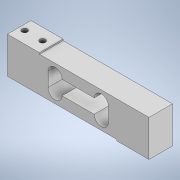
# Autodesk Inventor part: load_cell
Saved by Autodesk Inventor 2022.3 (Build 263350000, 350)
## iProperties
Created: 2022-01-31
Part Number: load_cell
Material: Generic
Document SubType Name: Modeling
Designer: Martijn
Density: 1 g/cm^3
Appearance: Default
Author: Martijn
Autodesk Inventor part; units mm, degrees
ref_plane "YZ Plane" through (0, 0, 0) normal (1, 0, 0) x (0, 1, 0)
ref_plane "XZ Plane" through (0, 0, 0) normal (0, 1, 0) x (-1, 0, 0)
ref_plane "XY Plane" through (0, 0, 0) normal (0, 0, 1) x (1, 0, 0)
sketch "Sketch1" plane through (0, 0, 0) normal (0, 0, 1) x (1, 0, 0)
  line L0 (0, 0) -> (150, 0)
  line L1 (150, 0) -> (150, 40)
  line L2 (150, 40) -> (0, 40)
  line L3 (0, 40) -> (0, 0)
  dimension "d0" = 40
  dimension "d1" = 150
  constraints: 8 end point, 2 parallel, 1 horizontal, 1 perpendicular
  measures "d0" distance of L2.end L0.start
  measures "d1" distance of L1.end L2.end
extrude "Extrusion1" add sketch "Sketch1" along normal blind 25
sketch "Sketch2" plane through (0, 0, 25) normal (0, 0, 1) x (1, 0, 0)
  arc A0 (58, 27.5) -> (43, 27.5) centre (50.5, 27.5) ccw
  line L0 (43, 27.5) -> (43, 12.5)
  arc A1 (43, 12.5) -> (58, 12.5) centre (50.5, 12.5) ccw
  line L1 (58, 27.5) -> (75, 27.5)
  line L2 (75, 27.5) -> (75, 12.5)
  line L3 (75, 12.5) -> (58, 12.5)
  line L4 (0, 0) -> (150, 0) projected
  line L5 (75, 0) -> (75, 12.5)
  dimension "d4" = 7.5
  dimension "d5" = 15
  dimension "d6" = 12.5
  dimension "d7" = 17
  dimension "d8" = 7.5
  constraints: 10 end point, 4 point on circle, 4 point on line, 2 centre point, 2 perpendicular, 1 collinear, 1 horizontal, 1 midpoint, 1 vertical
  measures "d4" radius of A0
  measures "d5" distance between parallel lines of L3 L1
  measures "d6" distance between parallel lines of L4 L3
  measures "d7" distance from line of L1.start L2
  measures "d8" radius of A1
extrude "Extrusion2" cut sketch "Sketch2" against normal blind 25
sketch "Sketch3" plane through (0, 40, 0) normal (0, 1, 0) x (1, 0, 0)
  circle A0 centre (5.8, -12.5) radius 3
  circle A1 centre (24.8, -12.5) radius 3
  line L0 (0, 0) -> (0, -25) projected
  line L1 (150, -25) -> (0, -25) projected
  dimension "d11" = 6
  dimension "d12" = 6
  dimension "d13" = 19
  dimension "d14" = 5.8
  dimension "d15" = 12.5
  dimension "d16" = 12.5
  constraints: 2 centre point
  measures "d11" diameter of A0
  measures "d12" diameter of A1
  measures "d13" distance of A1.centre A0.centre
  measures "d14" distance from line of L0 A0.centre
  measures "d15" distance from line of L1 A0.centre
  measures "d16" distance from line of L1 A1.centre
extrude "Extrusion3" cut sketch "Sketch3" against normal blind 13
mirror "Mirror1" about plane through (75, 27.5, 25) normal (-1, 0, 0) of "Extrusion2"
sketch "Sketch4" plane through (0, 0, 0) normal (0, -1, 0) x (1, 0, 0)
  circle A0 centre (144.2, 12.5) radius 3
  circle A1 centre (125.2, 12.5) radius 3
  line L0 (150, 0) -> (150, 25) projected
  line L1 (0, 0) -> (150, 0) projected
  dimension "d19" = 6
  dimension "d20" = 5.8
  dimension "d21" = 12.5
  dimension "d22" = 19
  dimension "d23" = 12.5
  constraints: 2 centre point, 1 equal radius
  measures "d19" diameter of A1
  measures "d20" distance from line of L0 A0.centre
  measures "d21" distance from line of L1 A0.centre
  measures "d22" distance of A1.centre A0.centre
  measures "d23" distance from line of L1 A1.centre
extrude "Extrusion4" cut sketch "Sketch4" against normal blind 13
sketch "Sketch5" plane through (0, 0, 25) normal (0, 0, 1) x (1, 0, 0)
  line L0 (150, 0) -> (150, 40) projected
  line L1 (150, 40) -> (34, 40)
  line L2 (34, 40) -> (34, 38.6)
  line L3 (34, 38.6) -> (150, 38.6)
  line L4 (150, 38.6) -> (150, 40)
  line L5 (0, 40) -> (0, 0) projected
  line L6 (0, 0) -> (116, 0)
  line L7 (116, 0) -> (116, 1.4)
  line L8 (116, 1.4) -> (0, 1.4)
  line L9 (0, 1.4) -> (0, 0)
  point P0 (34, 39.3)
  point P1 (116, 0.7)
  point P2 (0, 1.4)
  dimension "d26" = 1.4
  dimension "d27" = 34
  dimension "d28" = 34
  dimension "d29" = 1.4
  constraints: 16 end point, 4 parallel, 2 horizontal, 2 midpoint, 2 perpendicular
  measures "d26" distance of L1.end L2.end
  measures "d27" distance from line of L5 point (34, 39.3)
  measures "d28" distance from line of L0 point (116, 0.7)
  measures "d29" distance between parallel lines of L6 L8
extrude "Extrusion5" cut sketch "Sketch5" against normal blind 25
body "Solid1"
